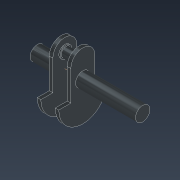
# Autodesk Inventor part: P015-Vilbrequin
Saved by Autodesk Inventor 2021.3 (Build 253353000, 353)
## iProperties
Created: 2022-04-01
Part Number: P015-Vilbrequin
Material: Iron, Gray
Document SubType Name: Modeling
Designer: remi
Density: 7.15 g/cm^3
Appearance: Iron Gray
Author: remi
Autodesk Inventor part; units mm, degrees
ref_plane "YZ Plane" through (0, 0, 0) normal (1, 0, 0) x (0, 1, 0)
ref_plane "XZ Plane" through (0, 0, 0) normal (0, 1, 0) x (-1, 0, 0)
ref_plane "XY Plane" through (0, 0, 0) normal (0, 0, 1) x (1, 0, 0)
sketch "Sketch2" plane through (0, 0, 0) normal (1, 0, 0) x (0, 1, 0)
  arc A0 (-20, 0) -> (20, 0) centre (0, 0) ccw
  line L0 (-20, 0) -> (-10, 0)
  line L1 (-10, 0) -> (-10, 25)
  line L2 (20, 0) -> (10, 0)
  line L3 (10, 0) -> (10, 25)
  arc A1 (10, 25) -> (-10, 25) centre (0, 25) ccw
  dimension "d1" = 20
  dimension "d2" = 25
  dimension "d3" = 20
  constraints: 8 end point, 4 horizontal alignment, 4 point on circle, 2 centre point, 2 horizontal, 2 perpendicular, 1 coincident, 1 collinear
  measures "d1" distance between parallel lines of L3 L1
  measures "d2" distance of L2.end L3.end
  measures "d3" radius of A0
extrude "Extrusion1" add sketch "Sketch2" along normal blind 3
sketch "Sketch3" plane through (3, 0, 0) normal (1, 0, 0) x (0, 0, -1)
  arc A0 (0, -20) -> (0, 20) centre (0, 0) ccw construction
  line L0 (0, 20) -> (0, 10) construction
  line L1 (0, 10) -> (-25, 10) construction
  arc A1 (-25, 10) -> (-25, -10) centre (-25, 0) ccw construction
  line L2 (-25, -10) -> (0, -10) construction
  line L3 (0, -10) -> (0, -20) construction
  circle A2 centre (-25, 0) radius 4
  dimension "d6" = 8
  constraints: 1 centre point, 1 coincident
  measures "d6" diameter of A2
extrude "Extrusion2" add sketch "Sketch3" along normal blind 12
sketch "Sketch4" plane through (15, 0, 25) normal (1, 0, 0) x (0, 0, -1)
  circle A0 centre (0, 0) radius 4 projected
  arc A1 (25, -20) -> (25, 20) centre (25, 0) ccw projected
  line L0 (25, 20) -> (25, 10) projected
  line L1 (25, 10) -> (0, 10) projected
  arc A2 (0, 10) -> (0, -10) centre (0, 0) ccw projected
  line L2 (0, -10) -> (25, -10) projected
  line L3 (25, -10) -> (25, -20) projected
extrude "Extrusion3" add sketch "Sketch4" along normal blind 3 contours A0 | L3 L2 A2 L1 L0 A1
sketch "Sketch5" plane through (3, 0, 0) normal (1, 0, 0) x (0, 0, -1)
  arc A0 (0, -20) -> (0, 20) centre (0, 0) ccw construction
  line L0 (0, -10) -> (0, -20) construction
  line L1 (-25, -10) -> (0, -10) construction
  arc A1 (-25, 10) -> (-25, -10) centre (-25, 0) ccw construction
  line L2 (0, 10) -> (-25, 10) construction
  line L3 (0, 20) -> (0, 10) construction
  circle A2 centre (-25, 0) radius 5
  circle A3 centre (-25, 0) radius 4 construction
  circle A4 centre (-25, 0) radius 4 construction
  dimension "d11" = 1
  constraints: 1 centre point, 1 coincident
  measures "d11" radial gap between concentric circles of A2 A3
extrude "Extrusion4" add sketch "Sketch5" along normal blind 1
sketch "Sketch6" plane through (15, 0, 25) normal (-1, 0, 0) x (0, 0, 1)
  line L0 (-25, 20) -> (-25, 10) construction
  arc A0 (-25, 20) -> (-25, -20) centre (-25, 0) ccw construction
  line L1 (-25, -10) -> (-25, -20) construction
  line L2 (0, -10) -> (-25, -10) construction
  arc A1 (0, -10) -> (0, 10) centre (0, 0) ccw construction
  line L3 (-25, 10) -> (0, 10) construction
  circle A2 centre (0, 0) radius 4 construction
  circle A3 centre (0, 0) radius 5
  dimension "d14" = 1
  constraints: 1 centre point, 1 coincident
  measures "d14" radial gap between concentric circles of A3 A2
extrude "Extrusion5" add sketch "Sketch6" along normal blind 1
sketch "Sketch7" plane through (0, 0, 0) normal (-1, 0, 0) x (0, 0, 1)
  line L0 (-31, 0) -> (46, 0) construction
  circle A0 centre (25, 0) radius 5 construction
  point P0 (0, 0)
  point P1 (0, 0)
  dimension "d24" = 25
  constraints: 1 point on line
  measures "d24" distance of point (0, 0) A0.centre
sketch "Sketch8" plane through (0, 0, 0) normal (-1, 0, 0) x (0, 0, 1)
  circle A0 centre (0, 0) radius 6
  dimension "d18" = 12
  constraints: 1 centre point, 1 coincident
  measures "d18" diameter of A0
extrude "Extrusion6" add sketch "Sketch8" along normal blind 20
sketch "Sketch9" plane through (18, 0, 25) normal (1, 0, 0) x (0, 0, -1)
  circle A0 centre (25, 0) radius 6
  dimension "d21" = 12
  constraints: 1 centre point, 1 coincident
  measures "d21" diameter of A0
extrude "Extrusion7" add sketch "Sketch9" along normal blind 50
equation "\"d12\" = d11"
equation "\"d15\" = d11"
body "Solid1"
